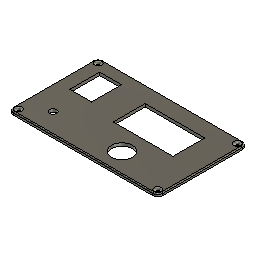
jumpy_usb_and_fan_mount (Autodesk Fusion 360 design; units mm, degrees)
part number: 2026-09-06-13-54-43-965
Autodesk Fusion 360 part; units mm, degrees
sketch "Sketch1" plane through (0, 0, 0) normal (0, 0, 1) x (1, 0, 0)
  line L0 (5, 0) -> (145, 0)
  line L1 (150, 5) -> (150, 85)
  line L2 (145, 90) -> (5, 90)
  line L3 (0, 85) -> (0, 5)
  line L4 (123.8126, 41.439) -> (63.8126, 41.439)
  line L5 (63.8126, 41.439) -> (63.8126, 73.439)
  line L6 (63.8126, 73.439) -> (123.8126, 73.439)
  line L7 (123.8126, 73.439) -> (123.8126, 41.439)
  line L8 (123.8126, 41.439) -> (63.8126, 73.439) construction
  line L9 (63.8126, 41.439) -> (123.8126, 73.439) construction
  line L10 (138.8126, 36.939) -> (48.8126, 36.939)
  line L11 (48.8126, 36.939) -> (48.8126, 77.939)
  line L12 (48.8126, 77.939) -> (138.8126, 77.939)
  line L13 (138.8126, 77.939) -> (138.8126, 36.939)
  line L14 (138.8126, 36.939) -> (48.8126, 77.939) construction
  line L15 (48.8126, 36.939) -> (138.8126, 77.939) construction
  line L16 (35.5073, 47.939) -> (13.5073, 47.939)
  line L17 (13.5073, 47.939) -> (13.5073, 77.939)
  line L18 (13.5073, 77.939) -> (35.5073, 77.939)
  line L19 (35.5073, 77.939) -> (35.5073, 47.939)
  line L20 (35.5073, 47.939) -> (13.5073, 77.939) construction
  line L21 (13.5073, 47.939) -> (35.5073, 77.939) construction
  circle A0 centre (24.5073, 20.2167) radius 3.5
  circle A1 centre (93.8126, 20.2167) radius 10.5
  arc A2 (5, 90) -> (0, 85) centre (5, 85) ccw
  arc A3 (150, 85) -> (145, 90) centre (145, 85) ccw
  arc A4 (145, 0) -> (150, 5) centre (145, 5) ccw
  arc A5 (0, 5) -> (5, 0) centre (5, 5) ccw
  circle A6 centre (5, 85) radius 1.5
  circle A7 centre (145, 85) radius 1.5
  circle A8 centre (145, 5) radius 1.5
  circle A9 centre (5, 5) radius 1.5
  point P0 (150, 0)
  point P1 (0, 90)
  point P2 (93.8126, 57.439)
  point P3 (93.8126, 57.439)
  point P4 (24.5073, 62.939)
  dimension "d1" = 150
  dimension "d2" = 90
  dimension "d3" = 60
  dimension "d4" = 32
  dimension "d5" = 90
  dimension "d6" = 41
  dimension "d7" = 22
  dimension "d8" = 30
  dimension "d9" = 7
  dimension "d10" = 21
  dimension "d13" = 5
  dimension "d14" = 5
  dimension "d15" = 5
  dimension "d16" = 5
  dimension "d17" = 3
  dimension "d18" = 3
  dimension "d19" = 3
  dimension "d20" = 3
  constraint horizontal L0
  constraint vertical L1
  constraint horizontal L2
  constraint vertical L3
  constraint horizontal L4
  constraint perpendicular L4 L5
  constraint parallel L4 L6
  constraint parallel L5 L7
  constraint coincident L8 P3
  constraint coincident L9 P3
  constraint horizontal L10
  constraint perpendicular L10 L11
  constraint parallel L10 L12
  constraint parallel L11 L13
  constraint coincident L14 P3
  constraint coincident L15 P3
  constraint coincident P3 P2
  constraint horizontal L16
  constraint perpendicular L16 L17
  constraint parallel L16 L18
  constraint parallel L17 L19
  constraint coincident L20 P4
  constraint coincident L21 P4
  constraint vertical P3 A1.centre
  constraint vertical P4 A0.centre
  constraint horizontal A0.centre A1.centre
  constraint coincident P1 L3
  constraint coincident P1 L2
  constraint tangent L3 A2
  constraint tangent L2 A2
  constraint tangent L2 A3
  constraint tangent L1 A3
  constraint coincident P0 L1
  constraint coincident P0 L0
  constraint tangent L1 A4
  constraint tangent L0 A4
  constraint coincident origin L0
  constraint coincident origin L3
  constraint tangent L0 A5
  constraint tangent L3 A5
  constraint concentric A2 A6
  constraint concentric A3 A7
  constraint concentric A4 A8
  constraint concentric A5 A9
  constraint collinear L12 L18
  measures "d1" distance of origin P0
  measures "d2" distance of origin P1
  measures "d3" distance of L5.end L6.end
  measures "d4" distance of L4.end L5.end
  measures "d5" distance of L11.end L12.end
  measures "d6" distance of L10.end L11.end
  measures "d7" distance of L17.end L18.end
  measures "d8" distance of L16.end L17.end
  measures "d9" diameter of A0
  measures "d10" diameter of A1
  measures "d13" radius of A2
  measures "d14" radius of A3
  measures "d15" radius of A4
  measures "d16" radius of A5
  measures "d17" diameter of A6
  measures "d18" diameter of A7
  measures "d19" diameter of A8
  measures "d20" diameter of A9
extrude "Extrude3" add sketch "Sketch1" along normal blind 3 contours L0 L1 L2 L3 A2 A3 A4 A5 | L10 L11 L12 L13
fillet "Fillet1" radius 2 4 edges at (3.6015, 85.5424, 3) (143.6015, 85.5424, 3) (143.6015, 5.5424, 3) (3.6015, 5.5424, 3)
fillet "Fillet2" radius 1 8 edges at (75, 0, 3) (148.5355, 1.4645, 3) (150, 45, 3) (148.5355, 88.5355, 3) (75, 90, 3) (1.4645, 88.5355, 3) (0, 45, 3) (1.4645, 1.4645, 3)
